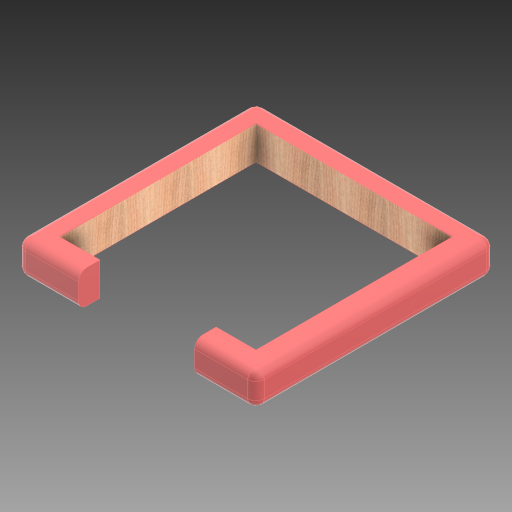
# Autodesk Inventor part: Bumper Template (WIP)
Saved by Autodesk Inventor 2023 (Build 270158000, 158)
## iProperties
RuleStatus: InUse
Created: 2022-12-12
Part Number: Bumper Template (WIP)
Material: Generic
Document SubType Name: Modeling
Designer: Cal
Density: 1 g/cm^3
Appearance: Smooth - Red
AfterAnyParamChange0: Bumper_Measurements
AfterAnyParamChange1: Bumper_Suppression
AfterAnyUserParamChange0: Bumper_Measurements
AfterAnyUserParamChange1: Bumper_Suppression
AfterFeatureSuppressionChange0: Bumper_Measurements
AfterFeatureSuppressionChange1: Bumper_Suppression
PartBodyChanged0: Bumper_Measurements
PartBodyChanged1: Bumper_Suppression
Author: Cal
Autodesk Inventor part; units mm, degrees
ref_plane "YZ Plane" through (0, 0, 0) normal (1, 0, 0) x (0, 1, 0)
ref_plane "XZ Plane" through (0, 0, 0) normal (0, 1, 0) x (-1, 0, 0)
ref_plane "XY Plane" through (0, 0, 0) normal (0, 0, 1) x (1, 0, 0)
sketch "Sketch1" plane through (0, 0, 0) normal (0, 1, 0) x (-1, 0, 0)
  line L0 (374.65, 374.65) -> (-374.65, 374.65)
  line L1 (-374.65, 374.65) -> (-374.65, -374.65)
  line L2 (-374.65, -374.65) -> (374.65, -374.65)
  line L3 (374.65, -374.65) -> (374.65, 374.65)
  line L4 (374.65, 374.65) -> (-374.65, -374.65) construction
  line L5 (-374.65, 374.65) -> (374.65, -374.65) construction
  line L6 (457.2, 457.2) -> (-457.2, 457.2)
  line L7 (-457.2, 457.2) -> (-457.2, -457.2)
  line L8 (-457.2, -457.2) -> (457.2, -457.2)
  line L9 (457.2, -457.2) -> (457.2, 457.2)
  line L10 (457.2, 457.2) -> (-457.2, -457.2) construction
  line L11 (-457.2, 457.2) -> (457.2, -457.2) construction
  point P0 (0, 0)
  dimension "d0" = 82.55
  dimension "d1" = 82.55
  dimension "d2" = 749.3
  dimension "d3" = 749.3
  constraints: 24 end point, 4 midpoint, 4 parallel, 2 horizontal, 2 perpendicular
  measures "d0" distance between parallel lines of L2 L8
  measures "d1" distance between parallel lines of L3 L9
  measures "d2" distance of L2.end L0.start
  measures "d3" distance of L0.start L0.end
extrude "Extrusion1" add sketch "Sketch1" along normal blind 127
fillet "Fillet1" radius 31.75 12 edges at (0, 127, 457.2) (0, 0, 457.2) (457.2, 63.5, 457.2) (457.2, 127, 0) (457.2, 0, 0) (457.2, 63.5, -457.2) (0, 127, -457.2) (-457.2, 127, 0) (-457.2, 63.5, 457.2) (0, 0, -457.2) (-457.2, 63.5, -457.2) (-457.2, 0, 0)
sketch "Bumper_Gaps" plane through (0, 127, 0) normal (0, 1, 0) x (1, 0, 0)
  line L0 (-222.25, -457.2) -> (222.25, -457.2)
  line L1 (222.25, -457.2) -> (222.25, -374.65)
  line L2 (222.25, -374.65) -> (-222.25, -374.65)
  line L3 (-222.25, -374.65) -> (-222.25, -457.2)
  line L4 (-222.25, -457.2) -> (222.25, -374.65) construction
  line L5 (222.25, -457.2) -> (-222.25, -374.65) construction
  line L6 (-457.2, -254) -> (-374.65, -254)
  line L7 (-374.65, -254) -> (-374.65, 254)
  line L8 (-374.65, 254) -> (-457.2, 254)
  line L9 (-457.2, 254) -> (-457.2, -254)
  line L10 (-457.2, -254) -> (-374.65, 254) construction
  line L11 (-374.65, -254) -> (-457.2, 254) construction
  line L12 (374.65, -254) -> (457.2, -254)
  line L13 (457.2, -254) -> (457.2, 254)
  line L14 (457.2, 254) -> (374.65, 254)
  line L15 (374.65, 254) -> (374.65, -254)
  line L16 (374.65, -254) -> (457.2, 254) construction
  line L17 (457.2, -254) -> (374.65, 254) construction
  line L18 (-374.65, -374.65) -> (-374.65, 374.65) projected
  line L19 (-457.2, 425.45) -> (-457.2, -425.45) projected
  line L20 (374.65, 374.65) -> (374.65, -374.65) projected
  line L21 (457.2, -425.45) -> (457.2, 425.45) projected
  line L22 (374.65, -374.65) -> (-374.65, -374.65) projected
  line L23 (-425.45, -457.2) -> (425.45, -457.2) projected
  line L24 (-196.85, 374.65) -> (196.85, 374.65)
  line L25 (196.85, 374.65) -> (196.85, 457.2)
  line L26 (196.85, 457.2) -> (-196.85, 457.2)
  line L27 (-196.85, 457.2) -> (-196.85, 374.65)
  line L28 (-196.85, 374.65) -> (196.85, 457.2) construction
  line L29 (196.85, 374.65) -> (-196.85, 457.2) construction
  line L30 (425.45, 457.2) -> (-425.45, 457.2) projected
  line L31 (-374.65, 374.65) -> (374.65, 374.65) projected
  point P0 (0, 0)
  point P1 (0, -415.925)
  point P2 (-415.925, 0)
  point P3 (415.925, 0)
  point P4 (0, 415.925)
  dimension "d15" = 444.5
  dimension "d16" = 393.7
  dimension "d17" = 508
  dimension "d18" = 508
  constraints: 48 end point, 8 collinear, 8 midpoint, 8 parallel, 4 horizontal, 4 perpendicular, 2 horizontal alignment, 2 vertical alignment
  measures "d15" distance between parallel lines of L1 L3
  measures "d16" distance between parallel lines of L25 L27
  measures "d17" distance between parallel lines of L14 L12
  measures "d18" distance between parallel lines of L8 L6
extrude "Front_Gap" cut sketch "Bumper_Gaps" against normal through all contours L3 L2 L1 L0
extrude "Back_Gap" [suppressed]
extrude "Left_Gap" [suppressed]
extrude "Right_Gap" [suppressed]
equation "\"d1\" = d0"
equation "\"d2\" = Length"
equation "\"d3\" = Width"
equation "\"d15\" = Front_Width"
equation "\"d16\" = Back_Width"
equation "\"d17\" = Left_Width"
equation "\"d18\" = Right_Width"
equation "\"Length\" = 749.3"
equation "\"Width\" = 749.3"
equation "\"Front_Width\" = 444.5"
equation "\"Back_Width\" = 393.7"
equation "\"Left_Width\" = 508"
equation "\"Right_Width\" = 508"
equation "\"Front_Edge\" = 152.4"
equation "\"Back_Edge\" = 152.4"
equation "\"Left_Edge\" = 152.4"
equation "\"Right_Edge\" = 152.4"
equation "\"FECalc\" = -0.5 * Front_Width + 0.5 * Width"
equation "\"BECalc\" = -0.5 * Back_Width + 0.5 * Width"
equation "\"LECalc\" = -0.5 * Left_Width + 0.5 * Length"
equation "\"RECalc\" = -0.5 * Right_Width + 0.5 * Length"
equation "\"FWCalc\" = Width - 2 * Front_Edge"
equation "\"BWCalc\" = Width - 2 * Back_Edge"
equation "\"LWCalc\" = Length - 2 * Left_Edge"
equation "\"RWCalc\" = Length - 2 * Right_Edge"
body "Solid1"
